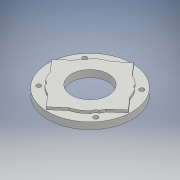
# Autodesk Inventor part: FilterHolderSmall
Saved by Autodesk Inventor 2017 (Build 210142000, 142)
## iProperties
Created: 2017-12-06
Part Number: FilterHolderSmall
Material: Generic
Document SubType Name: Modeling
Designer: Paolo
Density: 1 g/cm^3
Appearance: Default
Author: Paolo
Autodesk Inventor part; units mm, degrees
ref_plane "YZ Plane" through (0, 0, 0) normal (1, 0, 0) x (0, 1, 0)
ref_plane "XZ Plane" through (0, 0, 0) normal (0, 1, 0) x (-1, 0, 0)
sketch "Sketch1" plane through (0, 0, 0) normal (0, 0, 1) x (1, 0, 0)
  circle A0 centre (0, 0) radius 12.7 projected
  circle A1 centre (0, 0) radius 10.5 projected
  circle A2 centre (0, 0) radius 14.3
  dimension "d0" = 1.6
  constraints: 1 centre point
  measures "d0" radial gap between concentric circles of A0 A2
extrude "Extrusion1" add sketch "Sketch1" along normal blind 1.6 contours A0 | A2
sketch "Sketch2" plane through (0, 0, 0) normal (0, 0, -1) x (-1, 0, 0)
  circle A0 centre (0, 0) radius 12.7 projected
  circle A1 centre (0, 0) radius 14.3 projected
  circle A2 centre (0, 0) radius 13
  dimension "d3" = 0.3
  constraints: 1 centre point
  measures "d3" radial gap between concentric circles of A0 A2
extrude "Extrusion2" add sketch "Sketch2" along normal blind 6.3 contours A1
sketch "Sketch3" plane through (0, 0, -6.3) normal (0, 0, -1) x (-1, 0, 0)
  circle A0 centre (0, 0) radius 14.3
  circle A1 centre (19.874255, -0.376393) radius 1.05
  circle A2 centre (12.66567, 10.260688) radius 1
  circle A3 centre (-12.328513, 10.799987) radius 1.05
  circle A4 centre (-20.116437, 0.486485) radius 1.05
  circle A5 centre (-12.781524, -10.195126) radius 1.05
  circle A6 centre (12.212659, -10.734425) radius 1
  circle A7 centre (0, 0) radius 18.8
  circle A8 centre (0, 0) radius 13
  dimension "d6" = 4.5
  constraints: 1 centre point
  measures "d6" radial gap between concentric circles of A0 A7
ref_plane "Work Plane1" through (-47.73085, -37.950225, -7.3) normal (0, 0, 1) x (0.9997673, 0.0215719, 0)
extrude "Extrusion3" add sketch "Sketch3" along normal up to surface (1 mm away) contours A0 | A7
fillet "Fillet1" [suppressed]
sketch "Sketch4" plane through (0, 0, -6.3) normal (0, 0, 1) x (1, 0, 0)
  arc A0 (-13.212659, -10.734425) -> (-13.212659, -10.734425) centre (-12.212659, -10.734425) ccw
  circle A1 centre (-12.212659, -10.734425) radius 2.5
  circle A2 centre (12.781524, -10.195126) radius 1.05
  circle A3 centre (12.781524, -10.195126) radius 2.5
  circle A4 centre (12.328513, 10.799987) radius 1.05
  circle A5 centre (12.328513, 10.799987) radius 2.5
  circle A6 centre (-12.66567, 10.260688) radius 1
  circle A7 centre (-12.66567, 10.260688) radius 2.5
  circle A8 centre (-12.212659, -10.734425) radius 1
  point P0 (0, 0)
  dimension "d10" = 5
  dimension "d11" = 5
  dimension "d12" = 5
  dimension "d13" = 5
  constraints: 5 centre point, 5 coincident, 1 concentric
  measures "d10" diameter of A1
  measures "d11" diameter of A3
  measures "d12" diameter of A5
  measures "d13" diameter of A7
extrude "Extrusion4" cut sketch "Sketch4" along normal blind 8.05
move faces "Move1" translate (0, 0, -3) faces at (11.363899, 6.236801, 1.6)
move faces "Move2" translate (0, 0, -3.25) faces at (-12.47305, -4.813811, -1.4)
sketch "Sketch5" plane through (0, 0, -4.65) normal (0, 0, 1) x (0.9998882, 0.0149516, 0)
  circle A0 centre (0, 0) radius 13
  arc A1 (10.023349, 10.199141) -> (11.681375, 8.248362) centre (12.488611, 10.614449) ccw
  arc A2 (10.023349, 10.199141) -> (-10.023349, 10.199141) centre (0, 0) ccw
  arc A3 (-11.821855, 8.045728) -> (-10.023349, 10.199141) centre (-12.51084, 10.448913) ccw
  arc A4 (-11.821855, 8.045728) -> (-11.767717, -8.124705) centre (0, 0) ccw
  arc A5 (-9.880918, -10.337188) -> (-11.767717, -8.124705) centre (-12.37179, -10.550627) ccw
  arc A6 (-9.880918, -10.337188) -> (10.146802, -10.076329) centre (0, 0) ccw
  arc A7 (11.845743, -8.010516) -> (10.146802, -10.076329) centre (12.627662, -10.385091) ccw
  arc A8 (11.845743, -8.010516) -> (11.681375, 8.248362) centre (0, 0) ccw
extrude "Extrusion5" add sketch "Sketch5" along normal blind 1.5 contours A0 | A1 A8 A7 A6 A5 A4 A3 A2
sketch "Sketch7" plane through (0, 0, -7.3) normal (0, 0, -1) x (-1, 0, 0)
  line L0 (-18.345755, -1.197191) -> (-1.197191, 18.345755)
  line L1 (-1.197191, 18.345755) -> (18.345755, 1.197191)
  line L2 (18.345755, 1.197191) -> (1.197191, -18.345755)
  line L3 (1.197191, -18.345755) -> (-18.345755, -1.197191)
  circle A0 centre (-12.328513, 10.799987) radius 1.05
  circle A1 centre (12.212659, -10.734425) radius 1
  line L4 (-12.328513, 10.799987) -> (12.212659, -10.734425) construction
  point P0 (0, 0)
  point P1 (0, 0)
  dimension "d24" = 26
  constraints: 10 end point, 1 coincident, 1 perpendicular, 9 other
  measures "d24" distance of L1.end L0.end
extrude "Extrusion6" add sketch "Sketch7" against normal up to surface (3.15 mm away) from surface at -1 contours L0 L1 L2 L3
sketch "Sketch8" plane through (0, 0, -7.3) normal (0, 0, -1) x (-1, 0, 0)
  arc A0 (-11.556744, 8.422094) -> (-13.700703, 4.096431) centre (0, 0) ccw
  arc A1 (-11.556744, 8.422094) -> (-9.869735, 10.347866) centre (-12.328513, 10.799987) ccw
  arc A2 (-5.842243, 13.052134) -> (-9.869735, 10.347866) centre (0, 0) ccw
  line L0 (-1.197191, 18.345755) -> (-5.842243, 13.052134)
  line L1 (4.096431, 13.700703) -> (-1.197191, 18.345755)
  arc A3 (10.174722, 10.048136) -> (4.096431, 13.700703) centre (0, 0) ccw
  arc A4 (10.174722, 10.048136) -> (11.94083, 7.868073) centre (12.66567, 10.260688) ccw
  arc A5 (13.052134, 5.842243) -> (11.94083, 7.868073) centre (0, 0) ccw
  line L2 (18.345755, 1.197191) -> (13.052134, 5.842243)
  line L3 (13.700703, -4.096431) -> (18.345755, 1.197191)
  arc A6 (11.644925, -8.299743) -> (13.700703, -4.096431) centre (0, 0) ccw
  arc A7 (11.644925, -8.299743) -> (9.725256, -10.483768) centre (12.212659, -10.734425) ccw
  arc A8 (5.842243, -13.052134) -> (9.725256, -10.483768) centre (0, 0) ccw
  line L4 (1.197191, -18.345755) -> (5.842243, -13.052134)
  line L5 (-4.096431, -13.700703) -> (1.197191, -18.345755)
  arc A9 (-10.296324, -9.923492) -> (-4.096431, -13.700703) centre (0, 0) ccw
  arc A10 (-10.296324, -9.923492) -> (-11.964189, -7.832508) centre (-12.781524, -10.195126) ccw
  arc A11 (-13.052134, -5.842243) -> (-11.964189, -7.832508) centre (0, 0) ccw
  line L6 (-18.345755, -1.197191) -> (-13.052134, -5.842243)
  line L7 (-13.700703, 4.096431) -> (-18.345755, -1.197191)
  point P0 (0, 0)
extrude "Extrusion7" cut sketch "Sketch8" against normal up to surface (1 mm away)
sketch "Sketch9" plane through (0, 0, -6.3) normal (0, 0, 1) x (1, 0, 0)
  circle A0 centre (0, 0) radius 18.8
  circle A1 centre (12.781524, -10.195126) radius 1.05
  circle A2 centre (-12.66567, 10.260688) radius 1
  circle A3 centre (-12.212659, -10.734425) radius 1
  circle A4 centre (12.328513, 10.799987) radius 1.05
  line L0 (13.700703, 4.096431) -> (18.345755, -1.197191)
  line L1 (18.345755, -1.197191) -> (13.052134, -5.842243)
  arc A5 (11.964189, -7.832508) -> (13.052134, -5.842243) centre (0, 0) ccw
  arc A6 (11.964189, -7.832508) -> (10.296324, -9.923492) centre (12.781524, -10.195126) ccw
  arc A7 (4.096431, -13.700703) -> (10.296324, -9.923492) centre (0, 0) ccw
  line L2 (4.096431, -13.700703) -> (-1.197191, -18.345755)
  line L3 (-1.197191, -18.345755) -> (-5.842243, -13.052134)
  arc A8 (-9.725256, -10.483768) -> (-5.842243, -13.052134) centre (0, 0) ccw
  arc A9 (-9.725256, -10.483768) -> (-11.644925, -8.299743) centre (-12.212659, -10.734425) ccw
  arc A10 (-13.700703, -4.096431) -> (-11.644925, -8.299743) centre (0, 0) ccw
  line L4 (-13.700703, -4.096431) -> (-18.345755, 1.197191)
  line L5 (-18.345755, 1.197191) -> (-13.052134, 5.842243)
  arc A11 (-11.94083, 7.868073) -> (-13.052134, 5.842243) centre (0, 0) ccw
  arc A12 (-11.94083, 7.868073) -> (-10.174722, 10.048136) centre (-12.66567, 10.260688) ccw
  arc A13 (-4.096431, 13.700703) -> (-10.174722, 10.048136) centre (0, 0) ccw
  line L6 (-4.096431, 13.700703) -> (1.197191, 18.345755)
  line L7 (1.197191, 18.345755) -> (5.842243, 13.052134)
  arc A14 (9.869735, 10.347866) -> (5.842243, 13.052134) centre (0, 0) ccw
  arc A15 (9.869735, 10.347866) -> (11.556744, 8.422094) centre (12.328513, 10.799987) ccw
  arc A16 (13.700703, 4.096431) -> (11.556744, 8.422094) centre (0, 0) ccw
extrude "Extrusion8" add sketch "Sketch9" along normal blind 2
sketch "Sketch10" plane through (0, 0, -3.15) normal (0, 0, 1) x (0.9998882, 0.0149516, 0)
  circle A0 centre (0, 0) radius 8.287259
  constraints: 1 centre point, 1 coincident
extrude "Extrusion9" cut sketch "Sketch10" against normal blind 4
body "Solid1"
